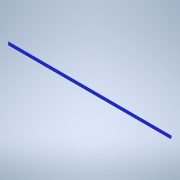
# Autodesk Inventor part: DR1-2000_On
Saved by Autodesk Inventor 2020.3 (Build 243373000, 373)
## iProperties
Part Number: DR1-2000_On
Material: PPS プラスチック
Catalog Web Link: www.cadenas.de
Description: Molded Flexible Racks (DR)-
Vendor: KHK
Document SubType Name: Modeling
Designer: partserver
Manufacturer: KHK
Mass: 10.1881 g
Surface Area: 92.613 cm^2
Volume: 6.22366 cm^3
Density: 1.637 g/cm^3
Appearance: 青 - 壁塗料 - 光沢
Category: PARTsolutions
Company: KHK
PSOL_IDENT_0: {$CADENAS_DATA\23d-libs\khk\racks\molded_flexible_racks_dr.prj},184 {VTYP=3D},{NB=DR1-2000_On},{LINA=
PSOL_IDENT_1: DR1-2000},{NN=Molded Flexible Racks (DR)},{DATE=10.04.2020 06:07:54},{GEOMDATE=26.02.2019 13:06:20},
PSOL_IDENT_2: {VERSION=},{LINEID=30},{WBVAR=TOOTH},{WBNUMERIC=}  {NB=DR1-2000_On},{LINA=DR1-2000},{KT=DUMMY},{CN=D
PSOL_IDENT_3: R1-2000},{M=1.0},{A=2000},{B=5.0},{B1=4},{C=4.3},{D=3.3},{E=2.0},{F=0.9},{G=4.9},{H=10},{ENT=632},{S=
PSOL_IDENT_4: R4},{WMF=R4001.WMF},{R=1.1},{TOOTH=On}
NB: DR1-2000_On
NN: Molded Flexible Racks (DR)
NBSYN: $CN._$TOOTH.
LINA: DR1-2000
CATALOG: KHK
CN: DR1-2000
M: 1
A: 2000
B: 5
B1: 4
C: 4.3
D: 3.3
E: 2
F: 0.9
G: 4.9
H: 10
ENT: 632
S: R4
TOOTH: On
SUPPLIER: KHK
ARTICLENO: DR1-2000_On
BOMINFO: DR1-2000
CREATOR: CADENAS GmbH
Title: DR1-2000
Author: Cadenas PARTsolutions
Autodesk Inventor part; units mm, degrees
ref_plane "YZ Plane" through (0, 0, 0) normal (1, 0, 0) x (0, 1, 0)
ref_plane "XZ Plane" through (0, 0, 0) normal (0, 1, 0) x (-1, 0, 0)
ref_plane "XY Plane" through (0, 0, 0) normal (0, 0, 1) x (1, 0, 0)
sketch "Sketch_1" plane through (0, 0, 0) normal (1, 0, 0) x (0, 0, -1)
  line L0 (-5, 0.9) -> (-5, 0)
  line L1 (-5, 0) -> (-2.45, 0)
  line L2 (-2.45, 0) -> (-2, 0.9)
  line L3 (-2, 0.9) -> (2, 0.9)
  line L4 (2, 0.9) -> (2.45, 0)
  line L5 (2.45, 0) -> (5, 0)
  line L6 (5, 0) -> (5, 0.9)
  arc A0 (5, 0.9) -> (3.9, 2) centre (3.9, 0.9) ccw
  line L7 (3.9, 2) -> (2.5, 2)
  line L8 (2.5, 2) -> (2, 4.3)
  line L9 (2, 4.3) -> (-2, 4.3)
  line L10 (-2, 4.3) -> (-2.5, 2)
  line L11 (-2.5, 2) -> (-3.9, 2)
  arc A1 (-3.9, 2) -> (-5, 0.9) centre (-3.9, 0.9) ccw
  constraints: 24 end point, 4 point on circle, 2 centre point
extrude "Extrusion1" add sketch "Sketch_1" along normal blind 550
sketch "Sketch_5" plane through (0, 0, 0) normal (0, 0, 1) x (1, 0, 0)
  line L0 (-1.1785, 4.3) -> (-0.3925, 2)
  line L1 (-0.3925, 2) -> (0.3925, 2)
  line L2 (0.3925, 2) -> (1.1785, 4.3)
  line L3 (1.1785, 4.3) -> (-1.1785, 4.3)
  constraints: 8 end point
extrude "Extrusion2" cut sketch "Sketch_5" along normal mid plane 5
pattern_linear "Rectangular Pattern1" count 641 spacing 3.1416 along (1, 0, 0) of "Extrusion2"
body "Solid1"
